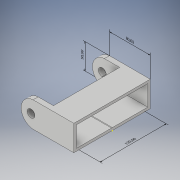
# Autodesk Inventor part: primer rotor
Saved by Autodesk Inventor 2019 (Build 230136000, 136)
## iProperties
Created: 2019-10-18
Part Number: primer rotor
Material: Genérico
Document SubType Name: Modeling
Designer: Josue
Density: 1 g/cm^3
Appearance: Valor por defecto
Author: Josue
Autodesk Inventor part; units mm, degrees
ref_plane "YZ Plane" through (0, 0, 0) normal (1, 0, 0) x (0, 1, 0)
ref_plane "XZ Plane" through (0, 0, 0) normal (0, 1, 0) x (-1, 0, 0)
sketch "Boceto1" plane through (0, 0, 0) normal (0, 1, 0) x (-1, 0, 0)
  line L0 (-25, 75) -> (25, 75)
  line L1 (25, 75) -> (25, -75)
  line L2 (25, -75) -> (-25, -75)
  line L3 (-25, -75) -> (-25, 75)
  line L4 (-25, 75) -> (25, -75) construction
  line L5 (25, 75) -> (-25, -75) construction
  point P0 (0, 0)
  dimension "d0" = 50
  dimension "d1" = 150
  constraints: 12 end point, 2 midpoint, 2 parallel, 1 horizontal, 1 perpendicular
  measures "d0" distance of L1.end L2.end
  measures "d1" distance of L0.end L1.end
extrude "Extrusión1" add sketch "Boceto1" along normal blind 50
sketch "Boceto2" plane through (25, 0, -75) normal (0, 0, -1) x (-1, 0, 0)
  line L0 (50, 50) -> (0, 50) projected
  line L1 (50, 50) -> (80, 50)
  line L2 (0, 0) -> (50, 0) projected
  line L3 (50, 0) -> (80, 0)
  arc A0 (80, 0) -> (80, 50) centre (78.3333, 25) ccw
  line L4 (50, 0) -> (50, 50) projected
  line L5 (50, 50) -> (50, 0)
  point P0 (25, 0)
  dimension "d4" = 30
  dimension "d5" = 30
  constraints: 6 end point, 2 horizontal, 2 point on circle, 1 centre point, 1 collinear
  measures "d4" distance of L0.start L1.end
  measures "d5" distance of L2.end L3.end
extrude "Extrusión2" add sketch "Boceto2" against normal blind 10
ref_plane "Plano de trabajo1" through (0, 25, 0) normal (0, 1, 0) x (1, 0, 0)
sketch "Boceto3" plane through (25, 0, -75) normal (0, 0, -1) x (-1, 0, 0)
  point P0 (25, 0)
  point P1 (84.2508, 24.8764)
hole "Agujero1" at (-59.2508, 24.8764, -75) direction (0, 0, 1) diameter 15 end through all
sketch "Boceto4" plane through (-25, 0, 75) normal (0, 0, 1) x (1, 0, 0)
  arc A0 (-30, 50) -> (-30, 0) centre (-28.3333, 25) ccw projected
  line L0 (0, 50) -> (-30, 50) projected
  line L1 (-30, 0) -> (0, 0) projected
  line L2 (0, 0) -> (0, 50) projected
  point P0 (25, 0)
extrude "Extrusión3" add sketch "Boceto4" against normal blind 10
sketch "Boceto5" plane through (25, 0, 75) normal (0, 0, 1) x (1, 0, 0)
  point P0 (-25, 0)
  point P1 (-83.9488, 24.8764)
hole "Agujero2" at (-58.9488, 24.8764, 75) direction (0, 0, -1) diameter 15 end through all
sketch "Boceto6" plane through (25, 0, 75) normal (1, 0, 0) x (0, 0, -1)
  point P0 (75, 0)
shell "Vaciado1" thickness 5 removed faces 1 at (25, 16.6667, -25)
sketch "Boceto7" plane through (-25, 0, -65) normal (-1, 0, 0) x (0, 0, 1)
  point P0 (65, 0)
  point P1 (65.2039, 25.1019)
hole "Agujero3" at (-25, 25.1019, 0.2039) direction (1, 0, 0) diameter 40.24 end through all
